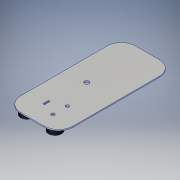
# Autodesk Inventor part: base
Saved by Autodesk Inventor 2018 (Build 220112000, 112)
## iProperties
Created: 2018-02-13
Part Number: base
Material: Aluminum 6061
Document SubType Name: Modeling
Designer: 238438
Density: 2.7 g/cm^3
Appearance: Aluminum - Flat
Author: 238438
Autodesk Inventor part; units mm, degrees
ref_plane "YZ Plane" through (0, 0, 0) normal (1, 0, 0) x (0, 1, 0)
ref_plane "XZ Plane" through (0, 0, 0) normal (0, 1, 0) x (-1, 0, 0)
ref_plane "XY Plane" through (0, 0, 0) normal (0, 0, 1) x (1, 0, 0)
sketch "Sketch1" plane through (0, 0, 0) normal (0, 1, 0) x (-1, 0, 0)
  line L0 (-25.2222, 0) -> (-46.0502, 0)
  line L1 (-58.7502, -12.7) -> (-58.7502, -88.8746)
  line L2 (-46.0502, -101.5746) -> (-25.2222, -101.5746)
  line L3 (-12.5222, -88.8746) -> (-12.5222, -12.7)
  arc A0 (-12.5222, -12.7) -> (-25.2222, 0) centre (-25.2222, -12.7) ccw
  arc A1 (-46.0502, 0) -> (-58.7502, -12.7) centre (-46.0502, -12.7) ccw
  arc A2 (-58.7502, -88.8746) -> (-46.0502, -101.5746) centre (-46.0502, -88.8746) ccw
  arc A3 (-25.2222, -101.5746) -> (-12.5222, -88.8746) centre (-25.2222, -88.8746) ccw
  circle A4 centre (-31.5722, -52.0446) radius 2.0066
  line L4 (-28.3972, -16.51) -> (-29.8704, -16.51)
  line L5 (-28.3972, -16.51) -> (-28.3972, -21.3868)
  line L6 (-28.3972, -21.3868) -> (-29.8704, -21.3868)
  line L7 (-29.8704, -21.3868) -> (-29.8704, -16.51)
  circle A5 centre (-40.9702, -12.7) radius 1.4097
  circle A6 centre (-40.9702, -25.4) radius 1.4097
  point P0 (0, 0)
  dimension "d1" = 101.5746
  dimension "d2" = 12.7
  dimension "d3" = 12.7
  dimension "d4" = 12.7
  dimension "d5" = 12.7
  dimension "d6" = 12.7
  dimension "d7" = 12.7
  dimension "d8" = 12.7
  dimension "d9" = 12.7
  dimension "d10" = 46.228
  dimension "d11" = 19.05
  dimension "d12" = 49.53
  dimension "d13" = 4.0132
  dimension "d14" = 1.4732
  dimension "d15" = 16.51
  dimension "d16" = 4.8768
  dimension "d17" = 15.875
  dimension "d18" = 12.7
  dimension "d19" = 17.78
  dimension "d20" = 12.7
  dimension "d21" = 2.8194
  dimension "d22" = 2.8194
  constraints: 16 end point, 8 point on circle, 7 centre point, 7 coincident, 4 tangent, 3 perpendicular, 2 horizontal, 2 parallel, 1 vertical
  measures "d1" distance between parallel lines of L0 L2
  measures "d2" distance from line of point (-46.05, -88.875) L1
  measures "d3" distance from line of L2 point (-46.05, -88.875)
  measures "d4" distance from line of L3 point (-25.222, -12.7)
  measures "d5" distance from line of L0 point (-25.222, -12.7)
  measures "d6" distance from line of L0 point (-46.05, -12.7)
  measures "d7" distance from line of L1 point (-46.05, -12.7)
  measures "d8" distance from line of L3 point (-25.222, -88.875)
  measures "d9" distance from line of L2 point (-25.222, -88.875)
  measures "d10" distance between parallel lines of L1 L3
  measures "d11" distance from line of L3 point (-31.572, -52.045)
  measures "d12" distance from line of L2 point (-31.572, -52.045)
  measures "d13" diameter of A4
  measures "d14" distance of L4.start L4.end
  measures "d15" distance between parallel lines of L0 L4
  measures "d16" distance of L4.start L5.end
  measures "d17" distance between parallel lines of L3 L5
  measures "d18" distance from line of L0 point (-40.97, -12.7)
  measures "d19" distance from line of L1 point (-40.97, -12.7)
  measures "d20" distance of point (-40.97, -12.7) point (-40.97, -25.4)
  measures "d21" diameter of A5
  measures "d22" diameter of A6
extrude "Extrusion1" add sketch "Sketch1" along normal blind 0.9779
sketch "Sketch2" plane through (0, 0, 0) normal (0, -1, 0) x (1, 0, 0)
  line L0 (58.7502, -88.8746) -> (58.7502, -12.7) projected
  line L1 (46.0502, 0) -> (25.2222, 0) projected
  circle A0 centre (47.9552, -7.62) radius 5.715
  line L2 (12.5222, -12.7) -> (12.5222, -88.8746) projected
  circle A1 centre (23.3172, -7.62) radius 5.715
  line L3 (25.2222, -101.5746) -> (46.0502, -101.5746) projected
  circle A2 centre (47.9552, -93.9546) radius 5.715
  circle A3 centre (23.3172, -93.9546) radius 5.715
  line L4 (29.8704, -16.51) -> (29.8704, -21.3868) projected
  line L5 (31.1404, -17.3228) -> (33.274, -17.3228)
  line L6 (33.274, -17.3228) -> (33.274, -22.1996)
  line L7 (33.274, -22.1996) -> (31.1404, -22.1996)
  line L8 (31.1404, -22.1996) -> (31.1404, -17.3228)
  line L9 (29.8704, -16.51) -> (28.3972, -16.51) projected
  line L10 (29.8704, -21.3868) -> (28.3972, -21.3868) projected
  line L11 (25.0952, -17.3228) -> (22.9616, -17.3228)
  line L12 (22.9616, -17.3228) -> (22.9616, -22.1996)
  line L13 (22.9616, -22.1996) -> (25.0952, -22.1996)
  line L14 (25.0952, -22.1996) -> (25.0952, -17.3228)
  point P0 (0, 0)
  dimension "d25" = 10.795
  dimension "d26" = 7.62
  dimension "d27" = 11.43
  dimension "d28" = 10.795
  dimension "d29" = 11.43
  dimension "d30" = 7.62
  dimension "d31" = 11.43
  dimension "d32" = 11.43
  dimension "d33" = 1.27
  dimension "d34" = 2.1336
  constraints: 16 end point, 4 centre point, 4 coincident, 2 parallel, 1 horizontal, 1 perpendicular
  measures "d25" distance from line of L0 point (47.955, -7.62)
  measures "d26" distance from line of L1 point (47.955, -7.62)
  measures "d27" diameter of A0
  measures "d28" distance from line of point (23.317, -7.62) L2
  measures "d29" diameter of A1
  measures "d30" distance from line of L3 point (47.955, -93.955)
  measures "d31" diameter of A2
  measures "d32" diameter of A3
  measures "d33" distance from line of L5.start L4
  measures "d34" distance of L6.end L7.end
extrude "Extrusion2" add sketch "Sketch2" along normal blind 5.08 contours A0 | A1 | A2 | A3
body "Solid1"
